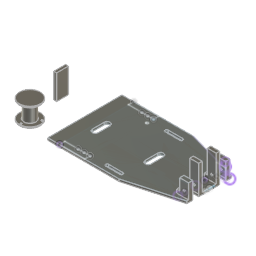
Chassis (Autodesk Fusion 360 design; units mm, degrees)
part number: 2026-03-16-02-33-25-626
Autodesk Fusion 360 part; units mm, degrees
sketch "Sketch1" plane through (0, 0, 0) normal (0, 0, 1) x (1, 0, 0)
  line L0 (0, 0) -> (100, 0)
  line L1 (59.344, 125) -> (0, 125)
  line L2 (0, 125) -> (0, 0)
  line L3 (190.267, 99.9338) -> (190.267, 25.0662)
  line L4 (190.267, 25.0662) -> (100, 0)
  line L5 (0, 62.5) -> (210, 62.5)
  line L6 (190.267, 62.5) -> (195, 62.5)
  line L7 (59.344, 125) -> (100, 125)
  line L8 (100, 125) -> (190.267, 99.9338)
  dimension "d1" = 100
  dimension "d2" = 125
  constraint horizontal L0
  constraint horizontal L1
  constraint vertical L2
  constraint coincident L0.start L2.end
  constraint perpendicular L1 L3
  constraint midpoint L2 L5.start
  constraint perpendicular L2 L5
  constraint midpoint L3 L6.start
  constraint perpendicular L3 L6
  constraint coincident L5 L6.start
  constraint parallel L1 L7
  measures "d1" distance of L0.start L0.end
  measures "d2" distance of L0.start L1.end
extrude "Extrude1" add sketch "Sketch1" along normal blind 4 makes body 1
sketch "Sketch2" plane through (0, 0, 4) normal (0, 0, 1) x (-1, 0, 0)
  line L0 (-100, -125) -> (0, -125)
  line L1 (0, -125) -> (0, 0)
  line L2 (0, 0) -> (-100, 0)
  line L3 (-100, 0) -> (-190.267, -25.0662)
  line L4 (-190.267, -25.0662) -> (-190.267, -99.9338)
  line L5 (-190.267, -25.0662) -> (-175.267, -25.0662)
  line L6 (-175.267, -25.0662) -> (-175.267, -35.0662)
  line L7 (-175.267, -35.0662) -> (-190.267, -35.0662)
  line L8 (-190.267, -35.0662) -> (-190.267, -25.0662)
  line L9 (-190.267, -45.0662) -> (-175, -45.0662)
  line L10 (-175, -45.0662) -> (-175, -50)
  line L11 (-175, -50) -> (-190.267, -50)
  line L12 (-190.267, -50) -> (-190.267, -45.0662)
  line L13 (-190.267, -99.9338) -> (-174.0176, -99.9338)
  line L14 (-174.0176, -99.9338) -> (-174.0176, -79.9997)
  line L15 (-174.0176, -79.9997) -> (-190.267, -79.9997)
  line L16 (-190.267, -79.9997) -> (-190.267, -99.9338)
  line L17 (-190.267, -69.9997) -> (-175, -69.9997)
  line L18 (-175, -69.9997) -> (-175, -60)
  line L19 (-175, -60) -> (-190.267, -60)
  line L20 (-190.267, -60) -> (-190.267, -69.9997)
  line L21 (-190.267, -99.9338) -> (-100, -125)
  dimension "d5" = 15
  dimension "d6" = 10
  dimension "d7" = 10
  dimension "d8" = 10
  constraint horizontal L5
  constraint vertical L6
  constraint horizontal L7
  constraint vertical L8
  constraint coincident L3.end L4.start
  constraint horizontal L9
  constraint vertical L10
  constraint horizontal L11
  constraint vertical L12
  constraint coincident L4 L9.start
  constraint horizontal L13
  constraint vertical L14
  constraint horizontal L15
  constraint vertical L16
  constraint coincident L4.end L13.start
  constraint horizontal L17
  constraint vertical L18
  constraint horizontal L19
  constraint vertical L20
  constraint coincident L4 L17.start
  measures "d5" distance of L3.end L5.end
  measures "d6" distance of L3.end L7.end
  measures "d7" distance of L7 L9
  measures "d8" distance of L15 L17
extrude "Extrude2" add sketch "Sketch2" along normal blind 25 contours L4 L13 L14 L15 L16 | L4 L17 L18 L19 L20 | L4 L5 L6 L7 L8 | L4 L9 L10 L11 L12 bodies 1
sketch "Sketch3" plane through (0, 0, 4) normal (0, 0, 1) x (-1, 0, 0)
  line L0 (-174.0176, -99.9338) -> (-190.267, -99.9338)
  line L1 (-100, -125) -> (0, -125)
  line L2 (0, -125) -> (0, 0)
  line L3 (0, 0) -> (-100, 0)
  line L4 (-100, 0) -> (-190.267, -25.0662)
  line L5 (-190.267, -25.0662) -> (-175.267, -25.0662)
  line L6 (-175.267, -25.0662) -> (-175.267, -35.0662)
  line L7 (-175.267, -35.0662) -> (-190.267, -35.0662)
  line L8 (-190.267, -35.0662) -> (-190.267, -45.0662)
  line L9 (-190.267, -45.0662) -> (-175, -45.0662)
  line L10 (-175, -45.0662) -> (-175, -50)
  line L11 (-175, -50) -> (-190.267, -50)
  line L12 (-190.267, -50) -> (-190.267, -60)
  line L13 (-190.267, -60) -> (-175, -60)
  line L14 (-175, -60) -> (-175, -69.9997)
  line L15 (-175, -69.9997) -> (-190.267, -69.9997)
  line L16 (-190.267, -69.9997) -> (-190.267, -79.9997)
  line L17 (-190.267, -79.9997) -> (-174.0176, -79.9997)
  line L18 (-174.0176, -79.9997) -> (-174.0176, -99.9338)
  line L19 (-190.267, -35.0662) -> (-175, -35.0662)
  line L20 (-175, -35.0662) -> (-175, -45.0662)
  line L21 (-175, -45.0662) -> (-190.267, -45.0662)
  line L22 (-190.267, -45.0662) -> (-190.267, -35.0662)
  line L23 (-190.267, -50) -> (-175, -50)
  line L24 (-175, -50) -> (-175, -60)
  line L25 (-175, -60) -> (-190.267, -60)
  line L26 (-190.267, -60) -> (-190.267, -50)
  line L27 (-190.267, -69.9997) -> (-174.0176, -69.9997)
  line L28 (-174.0176, -69.9997) -> (-174.0176, -79.9997)
  line L29 (-174.0176, -79.9997) -> (-190.267, -79.9997)
  line L30 (-190.267, -79.9997) -> (-190.267, -69.9997)
  line L31 (-190.267, -99.9338) -> (-100, -125)
  constraint horizontal L19
  constraint vertical L20
  constraint horizontal L21
  constraint vertical L22
  constraint coincident L9.end L10.start
  constraint coincident L7.end L8.start
  constraint horizontal L23
  constraint vertical L24
  constraint horizontal L25
  constraint vertical L26
  constraint coincident L13.end L14.start
  constraint coincident L11.end L12.start
  constraint horizontal L27
  constraint vertical L28
  constraint horizontal L29
  constraint vertical L30
  constraint coincident L17.end L18.start
  constraint coincident L15.end L16.start
extrude "Extrude3" cut sketch "Sketch3" against normal blind 5 contours L15 L16 L17 L27 L28 L29 L30 | L11 L12 L13 L23 L24 L25 L26 | L7 L8 L9 L19 L20 L21 L22 bodies 1
sketch "Sketch4" plane through (0, 0, 4) normal (0, 0, 1) x (-1, 0, 0)
  line L0 (-175, -35.0662) -> (-175, -45.0662)
  line L1 (-175, -45.0662) -> (-175, -50)
  line L2 (-175, -50) -> (-175, -60)
  line L3 (-175, -60) -> (-175, -69.9997)
  line L4 (-174.0176, -69.9997) -> (-174.0176, -79.9997)
  line L5 (-174.0176, -79.9997) -> (-174.0176, -99.9338)
  line L6 (-174.0176, -99.9338) -> (-190.267, -99.9338)
  line L7 (-100, -125) -> (0, -125)
  line L8 (0, -125) -> (0, 0)
  line L9 (0, 0) -> (-100, 0)
  line L10 (-100, 0) -> (-190.267, -25.0662)
  line L11 (-190.267, -25.0662) -> (-175.267, -25.0662)
  line L12 (-175.267, -25.0662) -> (-175.267, -35.0662)
  line L13 (0, -125) -> (-42.33, -125)
  line L14 (-42.33, -125) -> (-42.33, -116)
  line L15 (-42.33, -116) -> (0, -116)
  line L16 (0, -116) -> (0, -125)
  circle A0 centre (-42.33, -105) radius 1.6
  line L17 (-42.33, -116) -> (-32.33, -116)
  circle A1 centre (-32.33, -116) radius 1.6
  line L18 (-32.33, -116) -> (-22.33, -116)
  circle A2 centre (-22.33, -116) radius 1.6
  line L19 (0, 0) -> (-42.33, 0)
  line L20 (-42.33, 0) -> (-42.33, -9)
  line L21 (-42.33, -9) -> (0, -9)
  line L22 (0, -9) -> (0, 0)
  circle A3 centre (-42.33, -9) radius 1.6
  line L23 (-42.33, -9) -> (-32.33, -9)
  circle A4 centre (-32.33, -9) radius 1.6
  line L24 (-32.33, -9) -> (-22.33, -9)
  circle A5 centre (-22.33, -9) radius 1.6
  line L25 (-175, -69.9997) -> (-174.0176, -69.9997)
  line L26 (-190.267, -99.9338) -> (-100, -125)
  line L27 (-175.267, -35.0662) -> (-175, -35.0662)
  dimension "d13" = 42.33
  dimension "d14" = 9
  dimension "d15" = 3.2
  dimension "d16" = 10
  dimension "d17" = 3.2
  dimension "d18" = 10
  dimension "d19" = 3.2
  dimension "d20" = 42.33
  dimension "d21" = 9
  dimension "d22" = 3.2
  dimension "d23" = 10
  dimension "d24" = 3.2
  dimension "d25" = 10
  dimension "d26" = 3.2
  constraint horizontal L13
  constraint vertical L14
  constraint horizontal L15
  constraint vertical L16
  constraint coincident L7.end L8.start
  constraint coincident L14.end L15.start
  constraint perpendicular L14 L17
  constraint coincident L17.end A1.centre
  constraint parallel L15 L18
  constraint coincident L18.end A2.centre
  constraint horizontal L19
  constraint vertical L20
  constraint horizontal L21
  constraint vertical L22
  constraint coincident L8.end L9.start
  constraint coincident L20.end L21.start
  constraint parallel L21 L23
  constraint coincident L23.end A4.centre
  constraint parallel L21 L24
  constraint coincident L24.end A5.centre
  measures "d13" distance of L7.end L13.end
  measures "d14" distance of L7.end L15.end
  measures "d15" diameter of A0
  measures "d16" distance of L14.end L17.end
  measures "d17" diameter of A1
  measures "d18" distance of L17.end L18.end
  measures "d19" diameter of A2
  measures "d20" distance of L8.end L19.end
  measures "d21" distance of L8.end L21.end
  measures "d22" diameter of A3
  measures "d23" distance of L20.end L23.end
  measures "d24" diameter of A4
  measures "d25" distance of L23.end L24.end
  measures "d26" diameter of A5
extrude "Extrude4" cut sketch "Sketch4" against normal blind 13 contours L20 L21 A3 L23 | L20 L21 A3 L23 | L21 L24 A5 | L21 L24 A5 | L21 L23 A4 L24 | L21 L23 A4 L24 | L15 L18 A2 | L15 L18 A2 | L15 L17 A1 L18 | L15 L17 A1 L18 | A0 bodies 1
sketch "Sketch5" plane through (0, 0, 4) normal (0, 0, 1) x (-1, 0, 0)
  circle A0 centre (-22.33, -116) radius 1.6
  circle A1 centre (-22.33, -9) radius 1.6
  circle A2 centre (-32.33, -116) radius 1.6
  circle A3 centre (-42.33, -9) radius 1.6
  circle A4 centre (-32.33, -9) radius 1.6
  circle A5 centre (-42.33, -105) radius 1.6
  line L0 (-175, -35.0662) -> (-175, -45.0662)
  line L1 (-175, -45.0662) -> (-175, -50)
  line L2 (-175, -50) -> (-175, -60)
  line L3 (-175, -60) -> (-175, -69.9997)
  line L4 (-174.0176, -69.9997) -> (-174.0176, -79.9997)
  line L5 (-174.0176, -79.9997) -> (-174.0176, -99.9338)
  line L6 (-174.0176, -99.9338) -> (-190.267, -99.9338)
  line L7 (-100, -125) -> (0, -125)
  line L8 (0, -125) -> (0, 0)
  line L9 (0, 0) -> (-100, 0)
  line L10 (-100, 0) -> (-190.267, -25.0662)
  line L11 (-190.267, -25.0662) -> (-175.267, -25.0662)
  line L12 (-175.267, -25.0662) -> (-175.267, -35.0662)
  line L13 (-192.465, -55) -> (15.9238, -55)
  line L14 (-175, -69.9997) -> (-174.0176, -69.9997)
  line L15 (-190.267, -99.9338) -> (-100, -125)
  line L16 (-175.267, -35.0662) -> (-175, -35.0662)
  line L17 (-190.267, -25.0662) -> (-174.0176, -25.0662)
  line L18 (-174.0176, -25.0662) -> (-174.0176, -99.9338)
  line L19 (-174.0176, -99.9338) -> (-190.267, -99.9338)
  line L20 (-190.267, -99.9338) -> (-190.267, -25.0662)
  line L21 (-190.267, -25.0662) -> (-165, -25.0662)
  line L22 (-165, -25.0662) -> (-165, -100)
  line L23 (-165, -100) -> (-190.267, -100)
  line L24 (-190.267, -100) -> (-190.267, -25.0662)
  constraint perpendicular L2 L13
  constraint horizontal L17
  constraint vertical L18
  constraint horizontal L19
  constraint vertical L20
  constraint coincident L5.end L6.start
  constraint coincident L10.end L11.start
  constraint horizontal L21
  constraint vertical L22
  constraint horizontal L23
  constraint vertical L24
sketch "Sketch6" plane through (0, 0, 4) normal (0, 0, 1) x (-1, 0, 0)
  circle A0 centre (-42, -116) radius 1.6
  dimension "d29" = 3.2
  measures "d29" diameter of A0
extrude "Extrude5" add sketch "Sketch4" against normal blind 4 contours A0 bodies 1
sketch "Sketch7" plane through (0, 0, 4) normal (0, 0, 1) x (-1, 0, 0)
extrude "Extrude6" cut sketch "Sketch5" along normal blind 25 contours L0 L1 L2 L11 L12 L13 L16 L17 L20 L21 L24 | L2 L3 L4 L5 L6 L13 L14 L18 L19 L20 L24 | L13 L18 L21 L22 | L4 L5 L6 L13 L15 L18 L19 L22 L23 bodies 1
sketch "Sketch8" plane through (0, 0, 4) normal (0, 0, 1) x (-1, 0, 0)
  line L0 (-190, -25) -> (-170, -25)
  line L1 (-170, -25) -> (-170, -100)
  line L2 (-170, -100) -> (-190, -100)
  line L3 (-190, -100) -> (-190, -25)
  constraint horizontal L0
  constraint vertical L1
  constraint horizontal L2
  constraint vertical L3
extrude "Extrude7" add sketch "Sketch8" against normal blind 4 bodies 1
sketch "Sketch9" plane through (0, 0, 4) normal (0, 0, 1) x (-1, 0, 0)
  line L0 (-190, -79.9997) -> (-190.267, -79.9997)
  line L1 (-190.267, -79.9997) -> (-190.267, -99.9338)
  line L2 (-190.267, -99.9338) -> (-100, -125)
  line L3 (-100, -125) -> (0, -125)
  line L4 (0, -125) -> (0, 0)
  line L5 (0, 0) -> (-100, 0)
  line L6 (-100, 0) -> (-190.267, -25.0662)
  line L7 (-190.267, -25.0662) -> (-190.267, -35.0662)
  line L8 (-190.267, -35.0662) -> (-190, -35.0662)
  line L9 (-190, -35.0662) -> (-190, -45.0662)
  line L10 (-190, -45.0662) -> (-190.267, -45.0662)
  line L11 (-190.267, -45.0662) -> (-190.267, -50)
  line L12 (-190.267, -50) -> (-190, -50)
  line L13 (-190, -50) -> (-190, -60)
  line L14 (-190, -60) -> (-190.267, -60)
  line L15 (-190.267, -60) -> (-190.267, -69.9997)
  line L16 (-190.267, -69.9997) -> (-190, -69.9997)
  line L17 (-190, -69.9997) -> (-190, -79.9997)
  circle A0 centre (-32.33, -9) radius 1.6
  circle A1 centre (-42.33, -9) radius 1.6
  circle A2 centre (-32.33, -116) radius 1.6
  circle A3 centre (-22.33, -9) radius 1.6
  circle A4 centre (-22.33, -116) radius 1.6
  line L18 (-190.267, -25.0662) -> (-189.3194, -25.0662)
  line L19 (-189.3194, -25.0662) -> (-189.3194, -99.9338)
  line L20 (-189.3194, -99.9338) -> (-190.267, -99.9338)
  line L21 (-190.267, -99.9338) -> (-190.267, -25.0662)
  constraint horizontal L18
  constraint vertical L19
  constraint horizontal L20
  constraint vertical L21
  constraint coincident L6.end L7.start
extrude "Extrude8" cut sketch "Sketch9" against normal blind 5 contours L0 L1 L7 L8 L9 L10 L11 L12 L13 L14 L15 L16 L17 L18 L19 L20 L21 bodies 1
sketch "Sketch10" plane through (0, 0, 4) normal (0, 0, 1) x (-1, 0, 0)
  circle A0 centre (-22.33, -116) radius 1.6
  circle A1 centre (-22.33, -9) radius 1.6
  circle A2 centre (-32.33, -116) radius 1.6
  circle A3 centre (-42.33, -9) radius 1.6
  circle A4 centre (-32.33, -9) radius 1.6
  line L0 (-190.267, -25.0662) -> (-189.3194, -25.0662)
  line L1 (-189.3194, -25.0662) -> (-189.3194, -99.9338)
  line L2 (-189.3194, -99.9338) -> (-190.267, -99.9338)
  line L3 (-190.267, -99.9338) -> (-100, -125)
  line L4 (-100, -125) -> (0, -125)
  line L5 (0, -125) -> (0, 0)
  line L6 (0, 0) -> (-100, 0)
  line L7 (-100, 0) -> (-190.267, -25.0662)
  line L8 (-189.3194, -23.7428) -> (-204.6839, -23.7428)
  line L9 (-204.6839, -23.7428) -> (-204.6839, -108.4307)
  line L10 (-204.6839, -108.4307) -> (-189.3194, -108.4307)
  line L11 (-189.3194, -108.4307) -> (-189.3194, -23.7428)
  constraint horizontal L8
  constraint vertical L9
  constraint horizontal L10
  constraint vertical L11
extrude "Extrude9" cut sketch "Sketch10" against normal blind 4 contours L0 L7 L11 | L2 L3 L11 bodies 1
sketch "Sketch11" plane through (0, 0, 4) normal (0, 0, 1) x (-1, 0, 0)
extrude "Extrude10" cut sketch "Sketch6" against normal blind 4 bodies 1
extrude "Extrude11" add sketch "Sketch4" against normal blind 4 contours A0 bodies 1
sketch "Sketch12" plane through (0, 0, 4) normal (0, 0, 1) x (-1, 0, 0)
  circle A0 centre (-42, -116) radius 1.6
  dimension "d44" = 3.2
  measures "d44" diameter of A0
sketch "Sketch13" plane through (0, 0, 4) normal (0, 0, 1) x (-1, 0, 0)
  line L0 (-189.3194, -24.8031) -> (-174.3194, -24.8031)
  line L1 (-174.3194, -24.8031) -> (-174.3194, -34.8031)
  line L2 (-174.3194, -34.8031) -> (-189.3194, -34.8031)
  line L3 (-189.3194, -34.8031) -> (-189.3194, -24.8031)
  line L4 (-189.3194, -100.1969) -> (-174.3194, -100.1969)
  line L5 (-174.3194, -100.1969) -> (-174.3194, -90.1969)
  line L6 (-174.3194, -90.1969) -> (-189.3194, -90.1969)
  line L7 (-189.3194, -90.1969) -> (-189.3194, -100.1969)
  line L8 (-189.3194, -90.1969) -> (-189.3194, -80.1969)
  line L9 (-189.3194, -80.1969) -> (-174.3194, -80.1969)
  line L10 (-174.3194, -80.1969) -> (-174.3194, -70.1969)
  line L11 (-174.3194, -70.1969) -> (-189.3194, -70.1969)
  line L12 (-189.3194, -70.1969) -> (-189.3194, -80.1969)
  line L13 (-189.3194, -34.8031) -> (-189.3194, -44.8031)
  line L14 (-189.3194, -44.8031) -> (-174.3194, -44.8031)
  line L15 (-174.3194, -44.8031) -> (-174.3194, -54.8031)
  line L16 (-174.3194, -54.8031) -> (-189.3194, -54.8031)
  line L17 (-189.3194, -54.8031) -> (-189.3194, -44.8031)
  point P0 (-189.3194, -24.8031)
  point P1 (-189.3194, -100.1969)
  dimension "d45" = 15
  dimension "d46" = 10
  dimension "d47" = 15
  dimension "d48" = 10
  dimension "d49" = 10
  dimension "d50" = 15
  dimension "d51" = 10
  dimension "d52" = 10
  dimension "d53" = 15
  dimension "d54" = 10
  constraint horizontal L0
  constraint vertical L1
  constraint horizontal L2
  constraint vertical L3
  constraint coincident P0 L0.start
  constraint horizontal L4
  constraint vertical L5
  constraint horizontal L6
  constraint vertical L7
  constraint coincident P1 L4.start
  constraint perpendicular L6 L8
  constraint horizontal L9
  constraint vertical L10
  constraint horizontal L11
  constraint vertical L12
  constraint perpendicular L2 L13
  constraint horizontal L14
  constraint vertical L15
  constraint horizontal L16
  constraint vertical L17
  measures "d45" distance of P0 L0.end
  measures "d46" distance of P0 L2.end
  measures "d47" distance of P1 L4.end
  measures "d48" distance of P1 L6.end
  measures "d49" distance of L6.end L8.end
  measures "d50" distance of L8.end L9.end
  measures "d51" distance of L8.end L11.end
  measures "d52" distance of L2.end L13.end
  measures "d53" distance of L13.end L14.end
  measures "d54" distance of L13.end L16.end
extrude "Extrude12" add sketch "Sketch13" along normal blind 25 bodies 1
sketch "Sketch14" plane through (0, 0, 4) normal (0, 0, 1) x (-1, 0, 0)
sketch "Sketch15" plane through (0, 0, 4) normal (0, 0, 1) x (-1, 0, 0)
  line L0 (-189.3236, -34.8131) -> (-174.3236, -34.8131)
  line L1 (-174.3236, -34.8131) -> (-174.3236, -44.8131)
  line L2 (-174.3236, -44.8131) -> (-189.3236, -44.8131)
  line L3 (-189.3236, -44.8131) -> (-189.3236, -34.8131)
  line L4 (-189.3255, -80.1824) -> (-174.3255, -80.1824)
  line L5 (-174.3255, -80.1824) -> (-174.3255, -90.1824)
  line L6 (-174.3255, -90.1824) -> (-189.3255, -90.1824)
  line L7 (-189.3255, -90.1824) -> (-189.3255, -80.1824)
  dimension "d57" = 15
  dimension "d58" = 10
  dimension "d59" = 15
  dimension "d60" = 10
  constraint horizontal L0
  constraint vertical L1
  constraint horizontal L2
  constraint vertical L3
  constraint horizontal L4
  constraint vertical L5
  constraint horizontal L6
  constraint vertical L7
  measures "d57" distance of L0.start L0.end
  measures "d58" distance of L0.start L2.end
  measures "d59" distance of L4.start L4.end
  measures "d60" distance of L4.start L6.end
extrude "Extrude13" cut sketch "Sketch15" against normal blind 5 bodies 1
extrude "Extrude14" add 2 faces at (184.3194, 48.1364, 29) (179.3194, 76.8636, 29) along direction (0, 0, 1) blind 20 on bodies 1 bodies 1
extrude "Extrude15" add 1 faces at (0, 83.3333, 1.3333) along direction (-1, 0, 0) blind 20 on bodies 1 bodies 1
sketch "Sketch16" plane through (0, 0, 0) normal (0, 0, -1) x (1, 0, 0)
  line L0 (174.3255, -80.1824) -> (189.3194, -80.1824)
  line L1 (189.3194, -80.1824) -> (189.3194, -44.8131)
  line L2 (189.3194, -44.8131) -> (174.3236, -44.8131)
  line L3 (174.3236, -44.8131) -> (174.3236, -34.8131)
  line L4 (174.3236, -34.8131) -> (189.3194, -34.8131)
  line L5 (189.3194, -34.8131) -> (189.3194, -24.8031)
  line L6 (189.3194, -24.8031) -> (100, 0)
  line L7 (100, 0) -> (-20, 0)
  line L8 (-20, 0) -> (-20, -125)
  line L9 (-20, -125) -> (100, -125)
  line L10 (100, -125) -> (189.3194, -100.1969)
  line L11 (189.3194, -100.1969) -> (189.3194, -90.1824)
  line L12 (189.3194, -90.1824) -> (174.3255, -90.1824)
  line L13 (174.3255, -90.1824) -> (174.3255, -80.1824)
  circle A0 centre (42, -116) radius 1.6
  circle A1 centre (32.33, -9) radius 1.6
  circle A2 centre (42.33, -9) radius 1.6
  circle A3 centre (32.33, -116) radius 1.6
  circle A4 centre (22.33, -9) radius 1.6
  circle A5 centre (22.33, -116) radius 1.6
  circle A6 centre (149.7809, -62.4978) radius 17.5
  circle A7 centre (-65, -15) radius 17.5
  dimension "d67" = 35
  dimension "d68" = 35
  measures "d67" diameter of A6
  measures "d68" diameter of A7
extrude "Extrude16" add sketch "Sketch16" against normal blind 31 separate body contours A7 makes body 2
extrude "Extrude17" add 1 faces at (-70.7682, 15.8694, 31) along direction (0, 0, 1) blind 1 on bodies 2 bodies 2
sketch "Sketch17" plane through (0, 0, 0) normal (0, 0, -1) x (1, 0, 0)
  line L0 (174.3255, -80.1824) -> (189.3194, -80.1824)
  line L1 (189.3194, -80.1824) -> (189.3194, -44.8131)
  line L2 (189.3194, -44.8131) -> (174.3236, -44.8131)
  line L3 (174.3236, -44.8131) -> (174.3236, -34.8131)
  line L4 (174.3236, -34.8131) -> (189.3194, -34.8131)
  line L5 (189.3194, -34.8131) -> (189.3194, -24.8031)
  line L6 (189.3194, -24.8031) -> (100, 0)
  line L7 (100, 0) -> (-20, 0)
  line L8 (-20, 0) -> (-20, -125)
  line L9 (-20, -125) -> (100, -125)
  line L10 (100, -125) -> (189.3194, -100.1969)
  line L11 (189.3194, -100.1969) -> (189.3194, -90.1824)
  line L12 (189.3194, -90.1824) -> (174.3255, -90.1824)
  line L13 (174.3255, -90.1824) -> (174.3255, -80.1824)
  circle A0 centre (42, -116) radius 1.6
  circle A1 centre (32.33, -9) radius 1.6
  circle A2 centre (42.33, -9) radius 1.6
  circle A3 centre (32.33, -116) radius 1.6
  circle A4 centre (22.33, -9) radius 1.6
  circle A5 centre (22.33, -116) radius 1.6
  circle A6 centre (169.3194, -62.4978) radius 17.5
  dimension "d73" = 35
  dimension "d76" = 20
  measures "d73" diameter of A6
  measures "d76" distance of L1 A6.centre
extrude "Extrude18" cut sketch "Sketch17" against normal blind 1 contours A6 bodies 1
sketch "Sketch18" plane through (0, 0, 0) normal (0, 0, -1) x (1, 0, 0)
  circle A0 centre (-65, -15) radius 17.5
  line L0 (-65, -15) -> (-65, 2.5)
  line L1 (-65, -15) -> (-65, 0)
  circle A1 centre (-65, 0) radius 1.5
  circle A2 centre (-77.9904, -22.5) radius 1.5
  circle A3 centre (-52.0096, -22.5) radius 1.5
  dimension "d77" = 3
  dimension "d79" = 360
  constraint coincident A0.centre L0.start
  constraint coincident A0 L0.end
  constraint vertical L0
  constraint coincident L0 L1.end
  constraint coincident L1.end A1.centre
  measures "d77" diameter of A1
extrude "Extrude19" cut sketch "Sketch18" against normal blind 10 contours L0 L1 A1 | L0 L1 A1 | A2 | A3 bodies 2
sketch "Sketch19" plane through (0, 0, 32) normal (0, 0, 1) x (-1, 0, 0)
  circle A0 centre (65, -15) radius 17.5
  circle A1 centre (65, -15) radius 10
  dimension "d82" = 20
  constraint concentric A0 A1
  measures "d82" diameter of A1
extrude "Extrude20" cut sketch "Sketch19" against normal blind 30 bodies 2
sketch "Sketch20" plane through (0, 0, 32) normal (0, 0, 1) x (-1, 0, 0)
  circle A0 centre (65, -15) radius 10
  circle A1 centre (65, -15) radius 17.5
  dimension "d85" = 35
  constraint concentric A0 A1
  measures "d85" diameter of A1
extrude "Extrude21" add sketch "Sketch20" against normal blind 2 bodies 2
sketch "Sketch21" plane through (0, 0, 4) normal (0, 0, 1) x (-1, 0, 0)
  line L0 (-190, -70) -> (-190, -55.4993)
  line L1 (70, -60) -> (65, -60)
  line L2 (65, -60) -> (65, -80)
  line L3 (65, -80) -> (70, -80)
  line L4 (70, -80) -> (70, -60)
  dimension "d88" = 5
  dimension "d89" = 20
  constraint vertical L0
  constraint horizontal L1
  constraint vertical L2
  constraint horizontal L3
  constraint vertical L4
  measures "d88" distance of L1.start L1.end
  measures "d89" distance of L1.start L3.end
extrude "Extrude22" add sketch "Sketch21" along normal blind 42 separate body makes body 3
sketch "Sketch22" plane through (0, 0, 4) normal (0, 0, 1) x (-1, 0, 0)
  line L0 (-15, -50) -> (-15, -70)
  arc A0 (-15, -70) -> (-5, -70) centre (-10, -70) ccw
  line L1 (-5, -70) -> (-5, -50)
  arc A1 (-5, -50) -> (-15, -50) centre (-10, -50) ccw
  line L2 (-10, -50) -> (-10, -70) construction
  line L3 (-105, -48.9762) -> (-105, -70)
  arc A2 (-105, -70) -> (-95, -70) centre (-100, -70) ccw
  line L4 (-95, -70) -> (-95, -48.9762)
  arc A3 (-95, -48.9762) -> (-105, -48.9762) centre (-100, -48.9762) ccw
  line L5 (-100, -48.9762) -> (-100, -70) construction
  line L6 (-70, -107.5) -> (-95, -107.5)
  arc A4 (-95, -107.5) -> (-95, -112.5) centre (-95, -110) ccw
  line L7 (-95, -112.5) -> (-70, -112.5)
  arc A5 (-70, -112.5) -> (-70, -107.5) centre (-70, -110) ccw
  line L8 (-67.5, -110) -> (-97.5, -110) construction
  line L9 (-70, -7.5) -> (-94.2261, -7.5)
  arc A6 (-94.2261, -7.5) -> (-94.2261, -12.5) centre (-94.2261, -10) ccw
  line L10 (-94.2261, -12.5) -> (-70, -12.5)
  arc A7 (-70, -12.5) -> (-70, -7.5) centre (-70, -10) ccw
  line L11 (-70, -10) -> (-94.2261, -10) construction
  dimension "d92" = 10
  dimension "d93" = 10
  dimension "d94" = 5
  dimension "d95" = 5
  constraint tangent L0 A0
  constraint tangent A0 L1
  constraint parallel L0 L1
  constraint tangent L1 A1
  constraint tangent L0 A1
  constraint vertical L2
  constraint tangent L3 A2
  constraint tangent A2 L4
  constraint parallel L3 L4
  constraint tangent L4 A3
  constraint tangent L3 A3
  constraint parallel L0 L5
  constraint tangent L6 A4
  constraint tangent A4 L7
  constraint parallel L6 L7
  constraint tangent L7 A5
  constraint tangent L6 A5
  constraint midpoint A5 L8.start
  constraint midpoint A4 L8.end
  constraint horizontal L8
  constraint tangent L9 A6
  constraint tangent A6 L10
  constraint parallel L9 L10
  constraint tangent L10 A7
  constraint tangent L9 A7
  constraint horizontal L11
  measures "d92" diameter of A0
  measures "d93" diameter of A2
  measures "d94" diameter of A4
  measures "d95" diameter of A6
extrude "Extrude23" cut sketch "Sketch22" against normal blind 70 bodies 1
sketch "Sketch23" plane through (0, 0, 4) normal (0, 0, 1) x (-1, 0, 0)
  line L0 (-105, -70) -> (-105, -48.9762)
  arc A0 (-95, -48.9762) -> (-105, -48.9762) centre (-100, -48.9762) ccw
  line L1 (-95, -48.9762) -> (-95, -70)
  arc A1 (-105, -70) -> (-95, -70) centre (-100, -70) ccw
  line L2 (-15, -70) -> (-15, -50)
  arc A2 (-5, -50) -> (-15, -50) centre (-10, -50) ccw
  line L3 (-5, -50) -> (-5, -70)
  arc A3 (-15, -70) -> (-5, -70) centre (-10, -70) ccw
  line L4 (-95, -107.5) -> (-70, -107.5)
  arc A4 (-70, -112.5) -> (-70, -107.5) centre (-70, -110) ccw
  line L5 (-70, -112.5) -> (-95, -112.5)
  arc A5 (-95, -107.5) -> (-95, -112.5) centre (-95, -110) ccw
  line L6 (-94.2261, -7.5) -> (-70, -7.5)
  arc A6 (-70, -12.5) -> (-70, -7.5) centre (-70, -10) ccw
  line L7 (-70, -12.5) -> (-94.2261, -12.5)
  arc A7 (-94.2261, -7.5) -> (-94.2261, -12.5) centre (-94.2261, -10) ccw
  circle A8 centre (-32.33, -9) radius 1.6
  circle A9 centre (-42.33, -9) radius 1.6
  circle A10 centre (-32.33, -116) radius 1.6
  circle A11 centre (-22.33, -9) radius 1.6
  circle A12 centre (-22.33, -116) radius 1.6
  circle A13 centre (-42, -116) radius 1.6
  line L8 (-174.3255, -80.1969) -> (-174.3255, -90.1824)
  line L9 (-174.3255, -90.1824) -> (-189.3194, -90.1824)
  line L10 (-189.3194, -90.1824) -> (-189.3194, -90.1969)
  line L11 (-189.3194, -90.1969) -> (-174.3194, -90.1969)
  line L12 (-174.3194, -90.1969) -> (-174.3194, -100.1969)
  line L13 (-174.3194, -100.1969) -> (-189.3194, -100.1969)
  line L14 (-189.3194, -100.1969) -> (-100, -125)
  line L15 (-100, -125) -> (20, -125)
  line L16 (20, -125) -> (20, 0)
  line L17 (20, 0) -> (-100, 0)
  line L18 (-100, 0) -> (-189.3194, -24.8031)
  line L19 (-189.3194, -24.8031) -> (-174.3194, -24.8031)
  line L20 (-174.3194, -24.8031) -> (-174.3194, -34.8031)
  line L21 (-174.3194, -34.8031) -> (-189.3194, -34.8031)
  line L22 (-189.3194, -34.8031) -> (-189.3194, -34.8131)
  line L23 (-189.3194, -34.8131) -> (-174.3236, -34.8131)
  line L24 (-174.3236, -34.8131) -> (-174.3236, -44.8031)
  line L25 (-174.3236, -44.8031) -> (-174.3194, -44.8031)
  line L26 (-174.3194, -44.8031) -> (-174.3194, -54.8031)
  line L27 (-174.3194, -54.8031) -> (-189.3194, -54.8031)
  line L28 (-189.3194, -54.8031) -> (-189.3194, -70.1969)
  line L29 (-189.3194, -70.1969) -> (-174.3194, -70.1969)
  line L30 (-174.3194, -70.1969) -> (-174.3194, -80.1969)
  line L31 (-174.3194, -80.1969) -> (-174.3255, -80.1969)
  point P0 (-174.3194, -54.8031)
  point P1 (-174.3194, -24.8031)
sketch "Sketch24" plane through (0, 0, 4) normal (0, 0, 1) x (-1, 0, 0)
sketch "Sketch25" plane through (0, 0, 4) normal (0, 0, 1) x (-1, 0, 0)
  line L0 (-190, -55) -> (-190, -70)
  line L1 (-190, -70) -> (-190, -62.5)
  dimension "d98" = 7.5
  constraint vertical L0
  constraint parallel L0 L1
  measures "d98" distance of L0.end L1.end
sketch "Sketch26" plane through (0, 0, 4) normal (0, 0, 1) x (-1, 0, 0)
  line L0 (-174.3254, -44.8074) -> (-169.3254, -44.8074)
  line L1 (-169.3254, -44.8074) -> (-169.3254, -34.8074)
  line L2 (-169.3254, -34.8074) -> (-174.3254, -34.8074)
  line L3 (-174.3254, -34.8074) -> (-174.3254, -44.8074)
  dimension "d99" = 5
  dimension "d100" = 10
  constraint horizontal L0
  constraint vertical L1
  constraint horizontal L2
  constraint vertical L3
  measures "d99" distance of L0.start L0.end
  measures "d100" distance of L0.start L2.end
extrude "Extrude24" add sketch "Sketch26" along normal blind 10 bodies 1
sketch "Sketch27" plane through (0, 0, 4) normal (0, 0, 1) x (-1, 0, 0)
  line L0 (-174, -90) -> (-169, -90)
  line L1 (-169, -90) -> (-169, -80)
  line L2 (-169, -80) -> (-174, -80)
  line L3 (-174, -80) -> (-174, -90)
  dimension "d103" = 5
  constraint horizontal L0
  constraint vertical L1
  constraint horizontal L2
  constraint vertical L3
  measures "d103" distance of L0.start L0.end
extrude "Extrude25" add sketch "Sketch27" along normal blind 10 bodies 1
sketch "Sketch28" plane through (0, 0, 29) normal (0, 0, 1) x (-1, 0, 0)
  line L0 (-189.3194, -34.8031) -> (-174.3194, -34.8031)
  line L1 (-174.3194, -34.8031) -> (-174.3194, -24.8031)
  line L2 (-174.3194, -24.8031) -> (-189.3194, -24.8031)
  line L3 (-189.3194, -24.8031) -> (-189.3194, -34.8031)
sketch "Sketch29" plane through (0, 0, 49) normal (0, 0, 1) x (-1, 0, 0)
  line L0 (-189.3194, -54.8031) -> (-174.3194, -54.8031)
  line L1 (-174.3194, -54.8031) -> (-174.3194, -44.8031)
  line L2 (-174.3194, -44.8031) -> (-189.3194, -44.8031)
  line L3 (-189.3194, -44.8031) -> (-189.3194, -54.8031)
  line L4 (-174.3194, -54.8031) -> (-189.3194, -54.8031)
  line L5 (-189.3194, -54.8031) -> (-189.3194, -50.8031)
  line L6 (-189.3194, -50.8031) -> (-174.3194, -50.8031)
  line L7 (-174.3194, -50.8031) -> (-174.3194, -54.8031)
  dimension "d106" = 4
  constraint horizontal L4
  constraint vertical L5
  constraint horizontal L6
  constraint vertical L7
  constraint coincident L0.end L1.start
  measures "d106" distance of L0.end L6.end
extrude "Extrude26" cut sketch "Sketch29" against normal blind 45 contours L0 L1 L3 L4 L5 L6 L7 bodies 1
sketch "Sketch30" plane through (0, 0, 29) normal (0, 0, 1) x (-1, 0, 0)
  line L0 (-189.3194, -24.8031) -> (-174.3194, -24.8031)
  line L1 (-174.3194, -24.8031) -> (-174.3194, -27.8031)
  line L2 (-174.3194, -27.8031) -> (-189.3194, -27.8031)
  line L3 (-189.3194, -27.8031) -> (-189.3194, -24.8031)
  point P0 (-189.3194, -24.8031)
  dimension "d109" = 15
  dimension "d110" = 3
  constraint horizontal L0
  constraint vertical L1
  constraint horizontal L2
  constraint vertical L3
  constraint coincident P0 L0.start
  measures "d109" distance of P0 L0.end
  measures "d110" distance of P0 L2.end
extrude "Extrude27" cut sketch "Sketch30" against normal blind 25 bodies 1
sketch "Sketch31" plane through (0, 0, 49) normal (0, 0, 1) x (-1, 0, 0)
  line L0 (-189.3194, -70.1969) -> (-189.3194, -80.1969)
  line L1 (-189.3194, -80.1969) -> (-174.3194, -80.1969)
  line L2 (-174.3194, -80.1969) -> (-174.3194, -70.1969)
  line L3 (-174.3194, -70.1969) -> (-189.3194, -70.1969)
  line L4 (-174.3194, -70.1969) -> (-189.3194, -70.1969)
  line L5 (-189.3194, -70.1969) -> (-189.3194, -74.1969)
  line L6 (-189.3194, -74.1969) -> (-174.3194, -74.1969)
  line L7 (-174.3194, -74.1969) -> (-174.3194, -70.1969)
  line L8 (-189.3194, -100.1969) -> (-174.3194, -100.1969)
  line L9 (-174.3194, -100.1969) -> (-174.3194, -97.1969)
  line L10 (-174.3194, -97.1969) -> (-189.3194, -97.1969)
  line L11 (-189.3194, -97.1969) -> (-189.3194, -100.1969)
  point P0 (-189.3194, -100.1969)
  dimension "d113" = 4
  dimension "d114" = 15
  dimension "d115" = 3
  constraint horizontal L4
  constraint vertical L5
  constraint horizontal L6
  constraint vertical L7
  constraint coincident L2.end L3.start
  constraint horizontal L8
  constraint vertical L9
  constraint horizontal L10
  constraint vertical L11
  constraint coincident P0 L8.start
  measures "d113" distance of L2.end L6.end
  measures "d114" distance of P0 L8.end
  measures "d115" distance of P0 L10.end
extrude "Extrude28" cut sketch "Sketch31" against normal blind 45 contours L0 L2 L3 L4 L5 L6 L7 | L8 L9 L10 L11 bodies 1
extrude "Extrude29" cut 2 faces at (172.3333, 83.3333, 14) (172.6568, 38.1393, 14) along direction (0, 0, -1) blind 4 on bodies 1 bodies 1
sketch "Sketch32" plane through (0, 97.1969, 0) normal (0, 1, 0) x (-1, 0, 0)
  line L0 (-174.3194, 29) -> (-189.3194, 29)
  line L1 (-189.3194, 29) -> (-189.3194, 4)
  line L2 (-189.3194, 4) -> (-174.3194, 4)
  line L3 (-174.3194, 4) -> (-174.3194, 29)
  line L4 (-189.3194, 4) -> (-181.8194, 4)
  line L5 (-189.3194, 14) -> (-189.3194, 4)
  circle A0 centre (-181.8194, 14) radius 1.6
  dimension "d120" = 10
  dimension "d121" = 3.2
  constraint horizontal L4
  constraint vertical L5
  constraint coincident L1.end L2.start
  measures "d120" distance of L1.end L5.start
  measures "d121" diameter of A0
extrude "Extrude30" cut sketch "Sketch32" against normal blind 100 contours A0 bodies 1
sketch "Sketch33" plane through (0, 0, 10) normal (0, 0, 1) x (-1, 0, 0)
  line L0 (-174, -80) -> (-174, -90)
  line L1 (-174, -90) -> (-169, -90)
  line L2 (-169, -90) -> (-169, -80)
  line L3 (-169, -80) -> (-174, -80)
extrude "Extrude31" cut sketch "Sketch33" 1 faces at (172.6568, 38.1393, 10) against normal blind 6 on bodies 1 bodies 1
sketch "Sketch34" plane through (0, 0, 4) normal (0, 0, 1) x (-1, 0, 0)
  line L0 (-189.3194, -97.1969) -> (-174.3194, -97.1969)
  line L1 (-174.3194, -90.1969) -> (-174.3194, -100.1969)
  line L2 (-174.3255, -90.1824) -> (-189.3194, -90.1824)
  line L3 (-174.3194, -97.1969) -> (-169.3194, -97.1969)
  line L4 (-169.3194, -97.1969) -> (-169.3194, -74.1969)
  line L5 (-169.3194, -74.1969) -> (-174.3194, -74.1969)
  line L6 (-174.3194, -74.1969) -> (-174.3194, -97.1969)
  point P0 (-174.0176, -79.9997)
  point P1 (-174.3255, -80.1969)
  point P2 (-174.3255, -90.1824)
  point P3 (-174.3194, -97.1969)
  point P4 (-174.3194, -74.1969)
  dimension "d126" = 5
  dimension "d127" = 23
  constraint horizontal L3
  constraint vertical L4
  constraint horizontal L5
  constraint vertical L6
  constraint coincident P3 L0.end
  measures "d126" distance of P3 L3.end
  measures "d127" distance of P3 P4
extrude "Extrude32" add sketch "Sketch34" along normal blind 6 bodies 1
ref_plane "WorkPlane1" through (179.3194, 62.4999, 26.5) normal (0, -1, 0) x (-1, 0, 0)
sketch "Sketch35" plane through (0, 0, 4) normal (0, 0, 1) x (-1, 0, 0)
  line L0 (-174.3194, -50.8031) -> (-169.3194, -50.8031)
  line L1 (-169.3194, -50.8031) -> (-169.3194, -27.8031)
  line L2 (-169.3194, -27.8031) -> (-174.3194, -27.8031)
  line L3 (-174.3194, -27.8031) -> (-174.3194, -50.8031)
  point P0 (-174.3194, -50.8031)
  point P1 (-174.3194, -27.8031)
  dimension "d131" = 5
  dimension "d132" = 23
  constraint horizontal L0
  constraint vertical L1
  constraint horizontal L2
  constraint vertical L3
  constraint coincident P0 L0.start
  measures "d131" distance of P0 L0.end
  measures "d132" distance of P0 P1
extrude "Extrude33" add sketch "Sketch35" along normal blind 6 bodies 1
sketch "Sketch36" plane through (0, 90.1824, 0) normal (0, -1, 0) x (1, 0, 0)
  line L0 (189.3194, 0) -> (189.3194, 4)
  line L1 (189.3194, 4) -> (174.3255, 4)
  line L2 (174.3255, 4) -> (174.3255, 0)
  line L3 (174.3255, 0) -> (189.3194, 0)
  line L4 (189.3194, 4) -> (189.3194, 29)
  line L5 (174.3255, 0) -> (189.3255, 0)
  line L6 (189.3255, 0) -> (189.3255, 20)
  line L7 (189.3255, 20) -> (174.3255, 20)
  line L8 (174.3255, 20) -> (174.3255, 0)
  dimension "d136" = 15
  dimension "d137" = 20
  constraint horizontal L5
  constraint vertical L6
  constraint horizontal L7
  constraint vertical L8
  constraint coincident L2.end L3.start
  measures "d136" distance of L2.end L5.end
  measures "d137" distance of L2.end L7.end
sketch "Sketch37" plane through (0, 62.4999, 0) normal (0, -1, 0) x (-1, 0, 0)
sketch "Sketch38" plane through (0, 97.1969, 0) normal (0, 1, 0) x (-1, 0, 0)
  circle A0 centre (-181.8194, 14) radius 1.6
  line L0 (-174.3194, 29) -> (-189.3194, 29)
  line L1 (-189.3194, 29) -> (-189.3194, 4)
  line L2 (-189.3194, 4) -> (-169.3194, 4)
  line L3 (-169.3194, 4) -> (-169.3194, 10)
  line L4 (-169.3194, 10) -> (-174.3194, 10)
  line L5 (-174.3194, 10) -> (-174.3194, 29)
  circle A1 centre (-181.8194, 14) radius 1.6
  point P0 (-189.3194, 0)
sketch "Sketch39" plane through (0, 97.1969, 0) normal (0, 1, 0) x (-1, 0, 0)
  point P0 (-189.3194, 0)
  point P1 (-181.8194, 14)
